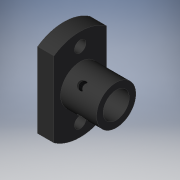
# Autodesk Inventor part: ATHC8-MB_b
Saved by Autodesk Inventor 2019 (Build 230136000, 136)
## iProperties
Created: 2022-12-26
Part Number: ATHC8-MB_b
Material: Generic
Catalog Web Link: www.cadenas.de
Description: STHCB, STHC, SSTHC, ATHC, BTHC_b-Shaft Supports - Bracket Shaped - Standard Type Drilled Mounting Hole - Compact Flange
Vendor: MISUMI
Document SubType Name: Modeling
Designer: psAdmin
Manufacturer: MISUMI
Mass: 2.43534 g
Surface Area: 20.4261 cm^2
Volume: 2.43534 cm^3
Density: 1 g/cm^3
Appearance: PSOLRGB-175-175-175
Category: PARTsolutions
Company: MISUMI
Title: ATHC8-MB
Author: Cadenas PARTsolutions
Comments: Shaft Supports - Bracket Shaped - Standard Type Drilled Mounting Hole - Compact Flange
PSOL_IDENT_0: {$CADENAS_DATA/23d-libs/misumi/metric/02_shaft_supports/ssthc/ssthc_body.prj},196 {VTYP=3D},{NB=ATHC
PSOL_IDENT_1: 8-MB_b},{LINA=ATHC8-MB},{NN=STHCB, STHC, SSTHC, ATHC, BTHC_b},{DATE=30.03.2018 01:12:54},{GEOMDATE=0
PSOL_IDENT_2: 6.10.2015 08:51:00},{VERSION=},{LINEID=50},{WBVAR=MAT,ST,M,ALT},{WBNUMERIC=}  {NB=ATHC8-MB_b},{LINA=
PSOL_IDENT_3: ATHC8-MB},{KT=DUMMY},{PN=ATHC8-MB},{TS=1},{TSALG= '1', 'Drilled Mounting Hole', '2', 'Tapped Mountin
PSOL_IDENT_4: g Hole' },{TYPE=ATHC},{MAT=AA},{MATA= '1018', 'SS400 Equivalent', '304', 'SUS304', 'AA'  , 'Aluminum
PSOL_IDENT_5: Alloy' },{MALG='M3'},{ST=CA},{ST0= 'CA', 'Clear Anodizing', 'BA', 'Black Anodizing' },{D=8},{THMD11='
PSOL_IDENT_6: M3','M4'},{THMD13='M4'},{THMD12='M3'},{DTOL=+0.015/0},{DX=8},{N=2.0},{L=16},{D1=12},{H=28},{T=5.0},{
PSOL_IDENT_7: LL=10},{M=M3},{THMD=3},{THMD1=M3},{THMD2=M3},{P=20},{K=22},{W=16},{P1=20},{F=0},{DD1=3.5},{DD11=3.5,
PSOL_IDENT_8: 4.5},{DD12=3.5,4.5},{M1=-},{M11=0},{ALT=MB},{ALTPN=-MB},{BM=3.0},{BL=3.0},{ANG=45}
NB: ATHC8-MB_b
NN: STHCB, STHC, SSTHC, ATHC, BTHC_b
NT: Shaft Supports - Bracket Shaped - Standard Type Drilled Mounting Hole - Compact Flange
NBSYN: $PN._b
LINA: ATHC8-MB
CATALOG: Misumi
PN: ATHC8-MB
MAT: Aluminum Alloy
ST: Clear Anodizing
D: 8
DTOL: +0.015/0
N: 2
L: 16
D1: 12
H: 28
T: 5
LL: 10
M: M3
W: 16
P1: 20
F: 0
DD1: 3.5
ALT: with MB (Hex Socket Set Screw Included)
SUPPLIER: MISUMI
ARTICLENO: ATHC8-MB_b
BOMINFO: ATHC8-MB
CREATOR: CADENAS GmbH
Autodesk Inventor part; units mm, degrees
sketch "Sketch_1" plane through (0, 0, 0) normal (0, 0, 1) x (1, 0, 0)
  line L0 (16, 0) -> (0, 0)
  line L1 (0, 4) -> (16, 4)
  line L2 (16, 4) -> (16, 6)
  line L3 (16, 6) -> (5, 6)
  line L4 (5, 6) -> (5, 14)
  line L5 (5, 14) -> (0, 14)
  line L6 (0, 14) -> (0, 4)
  constraints: 14 end point
revolve "Revolution1" add sketch "Sketch_1" angle 360 about axis through (16, 0, 0) along (1, 0, 0)
sketch "Sketch_19" plane through (10, 0, 0) normal (1, 0, 0) x (0, 0, -1)
  line L0 (-2.1213, 2.1213) -> (-4.2426, 4.2426)
  line L1 (-4.2426, 4.2426) -> (-3.182, 5.3033)
  line L2 (-3.182, 5.3033) -> (-3.182, 4.9208)
  line L3 (-3.182, 4.9208) -> (-1.2519, 2.9907)
  line L4 (-1.2519, 2.9907) -> (-2.1213, 2.1213)
  line L5 (-2.1213, 2.1213) -> (-4.2426, 4.2426)
  constraints: 12 end point
revolve "Revolution2" cut sketch "Sketch_19" angle 360 about axis through (10, 2.1213, 2.1213) along (0, -0.7071068, -0.7071068)
thread "Thread1" size "M3x0.5" class "6H" standard "ISO Metric profile" length 2.7295
sketch "Sketch_3" plane through (10, 0, 0) normal (1, 0, 0) x (0, 0, -1)
  line L0 (-2.1213, -2.1213) -> (-4.2426, -4.2426)
  line L1 (-4.2426, -4.2426) -> (-5.3033, -3.182)
  line L2 (-5.3033, -3.182) -> (-4.9208, -3.182)
  line L3 (-4.9208, -3.182) -> (-2.9907, -1.2519)
  line L4 (-2.9907, -1.2519) -> (-2.1213, -2.1213)
  line L5 (-2.1213, -2.1213) -> (-4.2426, -4.2426)
  constraints: 12 end point
revolve "Revolution3" cut sketch "Sketch_3" angle 360 about axis through (10, -2.1213, 2.1213) along (0, 0.7071068, -0.7071068)
thread "Thread2" size "M3x0.5" class "6H" standard "ISO Metric profile" length 2.7295
sketch "Sketch4" plane through (5, 0, 0) normal (1, 0, 0) x (0, 0, -1)
  point P0 (0, 10)
hole "Hole1" at (5, 10, 0) direction (-1, 0, 0) diameter 3.5 depth 5
sketch "Sketch5" plane through (0, 0, 0) normal (-1, 0, 0) x (0, 0, 1)
  point P0 (0, -10)
hole "Hole2" at (0, -10, 0) direction (1, 0, 0) diameter 3.5 depth 5
sketch "Sketch_4" plane through (0, 0, 0) normal (1, 0, 0) x (0, 1, 0)
  circle A0 centre (0, 0) radius 150
  line L0 (50, 8) -> (-50, 8)
  line L1 (-50, 8) -> (-50, -8)
  line L2 (-50, -8) -> (50, -8)
  line L3 (50, -8) -> (50, 8)
  constraints: 8 end point, 1 centre point
extrude "Extrusion1" cut sketch "Sketch_4" along normal blind 16
ref_plane "to_screw1_XY" through (10, -2.8284, 2.8284) normal (0, -0.7071068, 0.7071068) x (1, 0, 0)
ref_plane "to_screw1_YZ" through (10, -2.8284, 2.8284) normal (1, 0, 0) x (0, 0.7071068, 0.7071068)
ref_plane "to_screw1_ZX" through (10, -2.8284, 2.8284) normal (0, 0.7071068, 0.7071068) x (0, -0.7071068, 0.7071068)
ref_plane "to_screw2_XY" through (10, 2.8284, 2.8284) normal (0, 0.7071068, 0.7071068) x (1, 0, 0)
ref_plane "to_screw2_YZ" through (10, 2.8284, 2.8284) normal (1, 0, 0) x (0, 0.7071068, -0.7071068)
ref_plane "to_screw2_ZX" through (10, 2.8284, 2.8284) normal (0, 0.7071068, -0.7071068) x (0, 0.7071068, 0.7071068)
body "Solid1"
